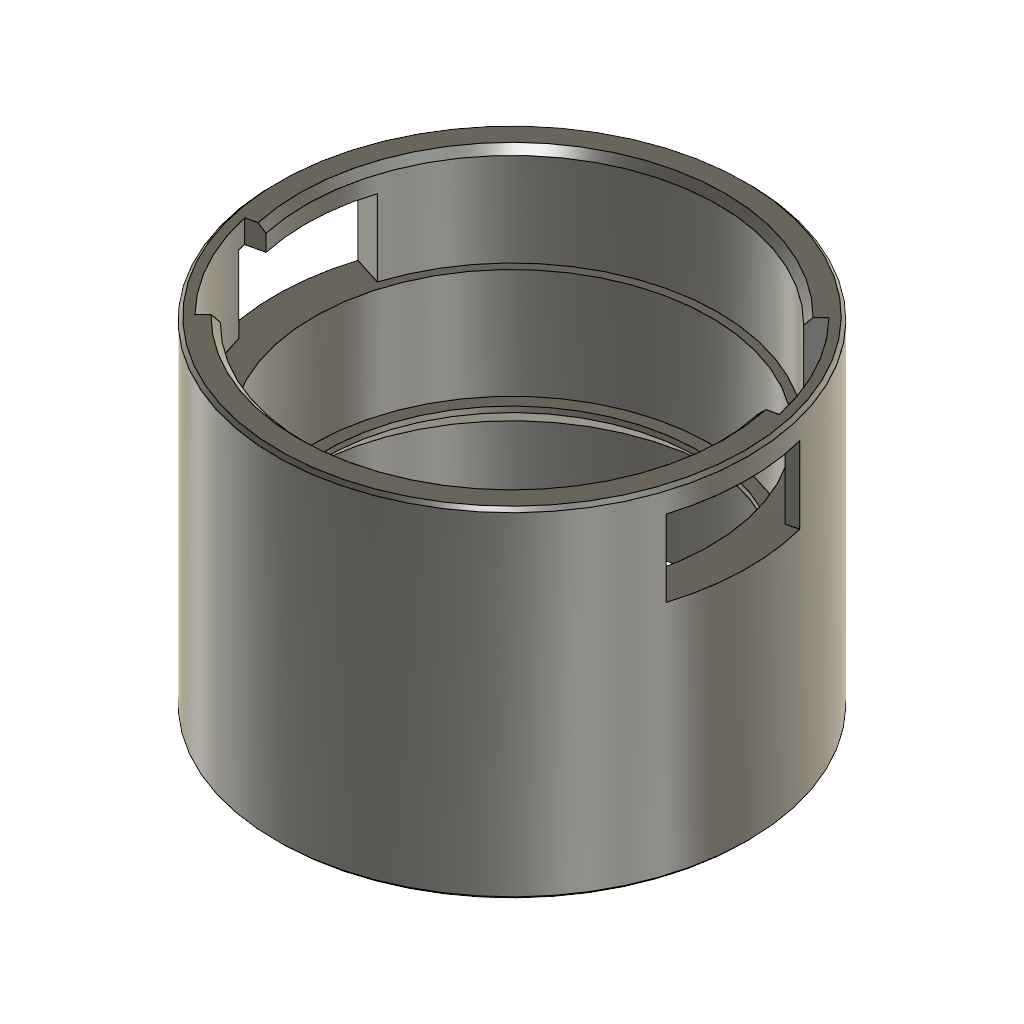
Part3_bayonet_flange (Autodesk Fusion 360 design; units mm, degrees)
part number: 2026-09-28-13-44-17-831
Autodesk Fusion 360 part; units mm, degrees
sketch "Sketch1" plane through (0, 0, 0) normal (0, 1, 0) x (1, 0, 0)
  line L0 (31.65, 0) -> (35, 0)
  line L1 (35, 0) -> (35.5, -0.5)
  line L2 (35.5, -0.5) -> (35.5, -50.5)
  line L3 (35.5, -50.5) -> (35, -51)
  line L4 (35, -51) -> (32, -51)
  line L5 (32, -51) -> (31, -50)
  line L6 (31, -50) -> (31, -36)
  line L7 (31, -36) -> (29.8, -36)
  line L8 (29.8, -36) -> (29.8, -19.5)
  line L9 (29.8, -19.5) -> (28, -19.5)
  line L10 (28, -19.5) -> (28, -18.65)
  line L11 (28, -18.65) -> (31.65, -15)
  line L12 (31.65, -15) -> (31.65, 0)
revolve "Revolve1" add sketch "Sketch1" angle 360 about axis through (0, 0, 1.75) along (0, 0, 1)
ref_plane "WorkPlane1" through (0, 0, 36) normal (0, 0, 1) x (1, 0, 0)
sketch "Windows" plane through (0, 0, 36) normal (0, 0, 1) x (1, 0, 0)
  arc A0 (27.6578, -8.7205) -> (28.0763, 7.261) centre (0, 0) ccw
  arc A1 (35.2875, -11.1261) -> (35.8215, 9.2641) centre (0, 0) ccw
  line L0 (27.6578, -8.7205) -> (35.2875, -11.1261)
  line L1 (28.0763, 7.261) -> (35.8215, 9.2641)
  arc A2 (-27.6578, 8.7205) -> (-28.0763, -7.261) centre (0, 0) ccw
  arc A3 (-35.2875, 11.1261) -> (-35.8215, -9.2641) centre (0, 0) ccw
  line L2 (-27.6578, 8.7205) -> (-35.2875, 11.1261)
  line L3 (-28.0763, -7.261) -> (-35.8215, -9.2641)
extrude "Windows (1)" cut sketch "Windows" along normal blind 11.5
ref_plane "WorkPlane2" through (0, 0, 36) normal (0, 0, 1) x (1, 0, 0)
sketch "Entry_grooves" plane through (0, 0, 36) normal (0, 0, 1) x (1, 0, 0)
  arc A0 (28.3126, 6.2767) -> (20.6843, 20.3264) centre (0, 0) ccw
  arc A1 (32.9012, 7.294) -> (24.0365, 23.6206) centre (0, 0) ccw
  line L0 (28.3126, 6.2767) -> (32.9012, 7.294)
  line L1 (20.6843, 20.3264) -> (24.0365, 23.6206)
  arc A2 (-28.3126, -6.2767) -> (-20.6843, -20.3264) centre (0, 0) ccw
  arc A3 (-32.9012, -7.294) -> (-24.0365, -23.6206) centre (0, 0) ccw
  line L2 (-28.3126, -6.2767) -> (-32.9012, -7.294)
  line L3 (-20.6843, -20.3264) -> (-24.0365, -23.6206)
extrude "Entry_grooves (1)" cut sketch "Entry_grooves" along normal blind 16
named bodies: "Part3_bayonet_flange"
